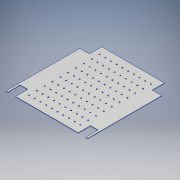
# Autodesk Inventor part: BK-BKT120-BasePlateLong_Ready
Saved by Autodesk Inventor 2017 (Build 210142000, 142)
## iProperties
Created: 2016-09-24
Part Number: BK-BKT120-BasePlateLong_Ready
Material: Aluminum 6061
Document SubType Name: Modeling
Designer: vslabsal
Density: 2.7 g/cm^3
Appearance: Aluminum - Flat
Author: vslabsal
Autodesk Inventor part; units mm, degrees
ref_plane "YZ Plane" through (0, 0, 0) normal (1, 0, 0) x (0, 1, 0)
ref_plane "XZ Plane" through (0, 0, 0) normal (0, 1, 0) x (-1, 0, 0)
ref_plane "XY Plane" through (0, 0, 0) normal (0, 0, 1) x (1, 0, 0)
sketch "Sketch1" plane through (0, 0, 0) normal (0, 0, 1) x (1, 0, 0)
  line L0 (270.51, 284.48) -> (-270.51, -284.48) construction
  line L1 (-270.51, 284.48) -> (270.51, -284.48) construction
  line L2 (-270.51, -284.48) -> (-257.81, -284.48)
  line L3 (-207.01, -284.48) -> (207.01, -284.48)
  line L4 (257.81, -284.48) -> (270.51, -284.48)
  line L5 (270.51, -284.48) -> (270.51, 203.2)
  line L6 (207.005, 284.48) -> (-207.015, 284.48)
  line L7 (-207.015, 206.375) -> (-207.015, 284.48)
  line L8 (-210.185, 203.2) -> (-270.51, 203.2)
  line L9 (-270.51, 203.2) -> (-270.51, -284.48)
  arc A0 (-210.185, 203.2) -> (-207.015, 206.375) centre (-210.19, 206.375) ccw
  line L10 (207.005, 284.48) -> (207.005, 206.375)
  line L11 (270.51, 203.2) -> (210.185, 203.2)
  arc A1 (207.005, 206.375) -> (210.185, 203.2) centre (210.18, 206.375) ccw
  line L12 (-257.81, -284.48) -> (-257.81, -206.375)
  line L13 (-207.01, -284.48) -> (-207.01, -206.375)
  arc A2 (-254.635, -203.2) -> (-257.81, -206.375) centre (-254.635, -206.375) ccw
  arc A3 (-207.01, -206.375) -> (-210.185, -203.2) centre (-210.185, -206.375) ccw
  line L14 (-254.635, -203.2) -> (-210.185, -203.2)
  line L15 (207.01, -284.48) -> (207.01, -206.375)
  line L16 (257.81, -284.48) -> (257.81, -206.375)
  arc A4 (210.185, -203.2) -> (207.01, -206.375) centre (210.185, -206.375) ccw
  arc A5 (257.81, -206.375) -> (254.635, -203.2) centre (254.635, -206.375) ccw
  line L17 (210.185, -203.2) -> (254.635, -203.2)
  point P0 (0, 0)
  point P1 (0, 0)
  dimension "d0" = 541.02
  dimension "d1" = 568.96
  dimension "d2" = 12.7
  dimension "d6" = 414.02
  dimension "d10" = 12.7
  dimension "d11" = 487.68
  dimension "d14" = 414.02
  dimension "d19" = 78.105
  dimension "d20" = 60.325
  dimension "d22" = 78.105
  dimension "d23" = 60.325
  dimension "d26" = 78.105
  dimension "d27" = 78.105
  dimension "d28" = 44.45
  dimension "d29" = 50.8
  dimension "d30" = 78.105
  dimension "d31" = 78.105
  constraints: 36 end point, 18 point on circle, 8 horizontal, 8 vertical, 6 centre point, 2 midpoint, 1 point on line, 1 tangent
  measures "d0" distance of L0.end L1.end
  measures "d1" distance of L1.start L0.end
  measures "d2" distance of L0.end L2.end
  measures "d6" distance of L3.start L3.end
  measures "d10" distance of L4.start L1.end
  measures "d11" distance of L1.end L5.end
  measures "d14" distance of L6.end L6.start
  measures "d19" distance of L7.start L6.end
  measures "d20" distance of L8.start L8.end
  measures "d22" distance of L6.start L10.end
  measures "d23" distance of L5.end L11.end
  measures "d26" distance of L3.start L13.end
  measures "d27" distance of L2.end L12.end
  measures "d28" distance of L14.start L14.end
  measures "d29" distance between parallel lines of L13 L12
  measures "d30" distance of L3.end L15.end
  measures "d31" distance of L4.start L16.end
extrude "Extrusion1" add sketch "Sketch1" along normal blind 3.175
sketch "Sketch2" plane through (0, 0, 3.175) normal (0, 0, 1) x (1, 0, 0)
  line L0 (-207.01, -206.375) -> (-207.01, -284.48) projected
  line L1 (-207.01, -284.48) -> (207.01, -284.48) projected
  line L2 (-270.51, 203.2) -> (-270.51, -284.48) projected
  circle A0 centre (-169.3718, -232.7564) radius 3.75
  circle A1 centre (-169.3718, -181.0327) radius 3.75
  circle A2 centre (-169.3718, -129.3091) radius 3.75
  circle A3 centre (-169.3718, -77.5855) radius 3.75
  circle A4 centre (-169.3718, -25.8618) radius 3.75
  circle A5 centre (-169.3718, 25.8618) radius 3.75
  circle A6 centre (-169.3718, 77.5855) radius 3.75
  circle A7 centre (-169.3718, 129.3091) radius 3.75
  circle A8 centre (-169.3718, 181.0327) radius 3.75
  circle A9 centre (-169.3718, 232.7564) radius 3.75
  circle A10 centre (-131.7336, -232.7564) radius 3.75
  circle A11 centre (-131.7336, -181.0327) radius 3.75
  circle A12 centre (-131.7336, -129.3091) radius 3.75
  circle A13 centre (-131.7336, -77.5855) radius 3.75
  circle A14 centre (-131.7336, -25.8618) radius 3.75
  circle A15 centre (-131.7336, 25.8618) radius 3.75
  circle A16 centre (-131.7336, 77.5855) radius 3.75
  circle A17 centre (-131.7336, 129.3091) radius 3.75
  circle A18 centre (-131.7336, 181.0327) radius 3.75
  circle A19 centre (-131.7336, 232.7564) radius 3.75
  circle A20 centre (-94.0955, -232.7564) radius 3.75
  circle A21 centre (-94.0955, -181.0327) radius 3.75
  circle A22 centre (-94.0955, -129.3091) radius 3.75
  circle A23 centre (-94.0955, -77.5855) radius 3.75
  circle A24 centre (-94.0955, -25.8618) radius 3.75
  circle A25 centre (-94.0955, 25.8618) radius 3.75
  circle A26 centre (-94.0955, 77.5855) radius 3.75
  circle A27 centre (-94.0955, 129.3091) radius 3.75
  circle A28 centre (-94.0955, 181.0327) radius 3.75
  circle A29 centre (-94.0955, 232.7564) radius 3.75
  circle A30 centre (-56.4573, -232.7564) radius 3.75
  circle A31 centre (-56.4573, -181.0327) radius 3.75
  circle A32 centre (-56.4573, -129.3091) radius 3.75
  circle A33 centre (-56.4573, -77.5855) radius 3.75
  circle A34 centre (-56.4573, -25.8618) radius 3.75
  circle A35 centre (-56.4573, 25.8618) radius 3.75
  circle A36 centre (-56.4573, 77.5855) radius 3.75
  circle A37 centre (-56.4573, 129.3091) radius 3.75
  circle A38 centre (-56.4573, 181.0327) radius 3.75
  circle A39 centre (-56.4573, 232.7564) radius 3.75
  circle A40 centre (-18.8191, -232.7564) radius 3.75
  circle A41 centre (-18.8191, -181.0327) radius 3.75
  circle A42 centre (-18.8191, -129.3091) radius 3.75
  circle A43 centre (-18.8191, -77.5855) radius 3.75
  circle A44 centre (-18.8191, -25.8618) radius 3.75
  circle A45 centre (-18.8191, 25.8618) radius 3.75
  circle A46 centre (-18.8191, 77.5855) radius 3.75
  circle A47 centre (-18.8191, 129.3091) radius 3.75
  circle A48 centre (-18.8191, 181.0327) radius 3.75
  circle A49 centre (-18.8191, 232.7564) radius 3.75
  circle A50 centre (18.8191, -232.7564) radius 3.75
  circle A51 centre (18.8191, -181.0327) radius 3.75
  circle A52 centre (18.8191, -129.3091) radius 3.75
  circle A53 centre (18.8191, -77.5855) radius 3.75
  circle A54 centre (18.8191, -25.8618) radius 3.75
  circle A55 centre (18.8191, 25.8618) radius 3.75
  circle A56 centre (18.8191, 77.5855) radius 3.75
  circle A57 centre (18.8191, 129.3091) radius 3.75
  circle A58 centre (18.8191, 181.0327) radius 3.75
  circle A59 centre (18.8191, 232.7564) radius 3.75
  circle A60 centre (56.4573, -232.7564) radius 3.75
  circle A61 centre (56.4573, -181.0327) radius 3.75
  circle A62 centre (56.4573, -129.3091) radius 3.75
  circle A63 centre (56.4573, -77.5855) radius 3.75
  circle A64 centre (56.4573, -25.8618) radius 3.75
  circle A65 centre (56.4573, 25.8618) radius 3.75
  circle A66 centre (56.4573, 77.5855) radius 3.75
  circle A67 centre (56.4573, 129.3091) radius 3.75
  circle A68 centre (56.4573, 181.0327) radius 3.75
  circle A69 centre (56.4573, 232.7564) radius 3.75
  circle A70 centre (94.0955, -232.7564) radius 3.75
  circle A71 centre (94.0955, -181.0327) radius 3.75
  circle A72 centre (94.0955, -129.3091) radius 3.75
  circle A73 centre (94.0955, -77.5855) radius 3.75
  circle A74 centre (94.0955, -25.8618) radius 3.75
  circle A75 centre (94.0955, 25.8618) radius 3.75
  circle A76 centre (94.0955, 77.5855) radius 3.75
  circle A77 centre (94.0955, 129.3091) radius 3.75
  circle A78 centre (94.0955, 181.0327) radius 3.75
  circle A79 centre (94.0955, 232.7564) radius 3.75
  circle A80 centre (131.7336, -232.7564) radius 3.75
  circle A81 centre (131.7336, -181.0327) radius 3.75
  circle A82 centre (131.7336, -129.3091) radius 3.75
  circle A83 centre (131.7336, -77.5855) radius 3.75
  circle A84 centre (131.7336, -25.8618) radius 3.75
  circle A85 centre (131.7336, 25.8618) radius 3.75
  circle A86 centre (131.7336, 77.5855) radius 3.75
  circle A87 centre (131.7336, 129.3091) radius 3.75
  circle A88 centre (131.7336, 181.0327) radius 3.75
  circle A89 centre (131.7336, 232.7564) radius 3.75
  circle A90 centre (169.3718, -232.7564) radius 3.75
  circle A91 centre (169.3718, -181.0327) radius 3.75
  circle A92 centre (169.3718, -129.3091) radius 3.75
  circle A93 centre (169.3718, -77.5855) radius 3.75
  circle A94 centre (169.3718, -25.8618) radius 3.75
  circle A95 centre (169.3718, 25.8618) radius 3.75
  circle A96 centre (169.3718, 77.5855) radius 3.75
  circle A97 centre (169.3718, 129.3091) radius 3.75
  circle A98 centre (169.3718, 181.0327) radius 3.75
  circle A99 centre (169.3718, 232.7564) radius 3.75
  point P0 (0, 0)
  dimension "d32" = 7.5
  dimension "d33" = 37.6382
  dimension "d34" = 51.7236
  dimension "d37" = 51.7236
  dimension "d40" = 37.6382
  constraints: 100 centre point, 1 horizontal, 1 vertical, 198 other
  measures "d32" diameter of A0
  measures "d33" distance from line of L0 A0.centre
  measures "d34" distance from line of L1 A0.centre
  measures "d37" distance of A0.centre A1.centre
  measures "d40" distance of A0.centre A10.centre
extrude "Extrusion2" cut sketch "Sketch2" against normal through all
body "Solid1"
